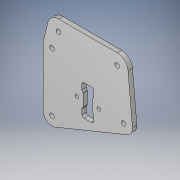
# Autodesk Inventor part: 上昇機構_内側板
Saved by Autodesk Inventor 2019.4 (Build 234330000, 330)
## iProperties
Created: 2021-12-04
Part Number: 上昇機構_内側板
Material: アルミニウム 6061
Document SubType Name: Modeling
Designer: 堀川皓史
Density: 2.7 g/cm^3
Appearance: アルミニウム - フラット
Mass: 27.3834 g
Surface Area: 78.2134 cm^2
Volume: 10.142 cm^3
Author: 堀川皓史
Autodesk Inventor part; units mm, degrees
ref_plane "YZ Plane" through (0, 0, 0) normal (1, 0, 0) x (0, 1, 0)
ref_plane "XZ Plane" through (0, 0, 0) normal (0, 1, 0) x (-1, 0, 0)
ref_plane "XY Plane" through (0, 0, 0) normal (0, 0, 1) x (1, 0, 0)
sketch "スケッチ1" plane through (0, 0, 0) normal (0, 0, 1) x (1, 0, 0)
  line L0 (-15, 61.4764) -> (15, 61.4764) construction
  line L1 (15, 61.4764) -> (15, -42.9448) construction
  line L2 (15, -42.9448) -> (-15, -42.9448) construction
  line L3 (-15, -42.9448) -> (-15, 61.4764) construction
  circle A0 centre (-24.5, 20) radius 9.5 construction
  circle A1 centre (24.5, 0) radius 9.5 construction
  circle A2 centre (-24.5, -20) radius 9.5 construction
  line L4 (-3, 9.5) -> (3, 9.5) construction
  line L5 (3, 9.5) -> (3, -9.5) construction
  line L6 (3, -9.5) -> (-3, -9.5) construction
  line L7 (-3, -9.5) -> (-3, 9.5) construction
  circle A3 centre (-7.5, 0) radius 1.25
  circle A4 centre (7.5, 0) radius 1.25
  circle A5 centre (-20, 32) radius 1.6
  circle A6 centre (20, 32) radius 1.6
  line L8 (-24.5, 20) -> (-24.5, -20) construction
  line L9 (-24.5, -20) -> (24.5, 0) construction
  line L10 (24.5, 0) -> (-24.5, 20) construction
  line L11 (-61.4764, 39.5) -> (49.785, 39.5) construction
  line L12 (49.785, 39.5) -> (49.785, 24.5) construction
  line L13 (49.785, 24.5) -> (-61.4764, 24.5) construction
  line L14 (-61.4764, 24.5) -> (-61.4764, 39.5) construction
  circle A7 centre (-24.5, 20) radius 1.6
  circle A8 centre (24.5, 0) radius 1.6
  circle A9 centre (-24.5, -20) radius 1.6
  arc A10 (-20, 39.5) -> (-27.2824, 33.7934) centre (-20, 32) ccw
  arc A11 (27.4674, 32.6985) -> (20, 39.5) centre (20, 32) ccw
  arc A12 (-30.3259, 21.4347) -> (-30.5, 20) centre (-24.5, 20) ccw
  arc A13 (-30.5, -20) -> (-22.2326, -25.5551) centre (-24.5, -20) ccw
  arc A14 (26.7674, -5.5551) -> (30.4739, 0.5588) centre (24.5, 0) ccw
  line L15 (-20, 39.5) -> (20, 39.5)
  line L16 (-27.2824, 33.7934) -> (-30.3259, 21.4347)
  line L17 (-30.5, 20) -> (-30.5, -20)
  line L18 (-22.2326, -25.5551) -> (26.7674, -5.5551)
  line L19 (30.4739, 0.5588) -> (27.4674, 32.6985)
  line L20 (-2.5, -10.5) -> (2.5, -10.5)
  line L21 (4, -9) -> (4, -5.6703)
  line L22 (2.5, 10.5) -> (-2.5, 10.5)
  line L23 (-3.1, 4) -> (-3.1, -4)
  line L24 (3.1, 4) -> (3.1, -4)
  line L25 (-4, -5.6703) -> (-4, -9)
  line L26 (4, 5.6703) -> (4, 9)
  arc A15 (-2.5, 10.5) -> (-4, 9) centre (-2.5, 9) ccw
  arc A16 (4, 9) -> (2.5, 10.5) centre (2.5, 9) ccw
  arc A17 (-4, -9) -> (-2.5, -10.5) centre (-2.5, -9) ccw
  arc A18 (2.5, -10.5) -> (4, -9) centre (2.5, -9) ccw
  line L27 (-4, 9) -> (-4, 5.6703)
  arc A19 (-4, 5.6703) -> (-3.325, 4.4176) centre (-2.5, 5.6703) ccw
  arc A20 (-3.1, 4) -> (-3.325, 4.4176) centre (-3.6, 4) ccw
  arc A21 (3.325, 4.4176) -> (4, 5.6703) centre (2.5, 5.6703) ccw
  arc A22 (3.325, 4.4176) -> (3.1, 4) centre (3.6, 4) ccw
  arc A23 (-3.325, -4.4176) -> (-4, -5.6703) centre (-2.5, -5.6703) ccw
  arc A24 (-3.325, -4.4176) -> (-3.1, -4) centre (-3.6, -4) ccw
  arc A25 (3.1, -4) -> (3.325, -4.4176) centre (3.6, -4) ccw
  arc A26 (4, -5.6703) -> (3.325, -4.4176) centre (2.5, -5.6703) ccw
  circle A27 centre (-24.5, 20) radius 4 construction
  point P0 (0, 0)
  dimension "d0" = 30
  dimension "d1" = 15
  dimension "d2" = 19
  dimension "d3" = 19
  dimension "d4" = 19
  dimension "d5" = 6
  dimension "d6" = 19
  dimension "d7" = 3
  dimension "d8" = 9.5
  dimension "d9" = 2.5
  dimension "d10" = 2.5
  dimension "d11" = 15
  dimension "d12" = 7.5
  dimension "d13" = 3.2
  dimension "d14" = 3.2
  dimension "d15" = 40
  dimension "d16" = 40
  dimension "d17" = 20
  dimension "d18" = 12
  dimension "d19" = 15
  dimension "d20" = 7.5
  dimension "d21" = 3.2
  dimension "d22" = 3.2
  dimension "d23" = 3.2
  dimension "d24" = 7.5
  dimension "d25" = 7.5
  dimension "d26" = 6
  dimension "d27" = 6
  dimension "d28" = 6
  dimension "d29" = 1
  dimension "d32" = 8
  dimension "d33" = 4
  dimension "d34" = 0.1
  dimension "d35" = 0.1
  dimension "d36" = 1
  dimension "d37" = 1
  dimension "d38" = 1
  dimension "d39" = 1.5
  dimension "d40" = 1
  dimension "d41" = 1.5
  dimension "d42" = 0.5
  dimension "d44" = 1
  dimension "d45" = 1.5
  dimension "d46" = 0.5
  dimension "d47" = 1.5
  dimension "d48" = 0.5
  dimension "d49" = 0.5
  dimension "d50" = 1.5
  dimension "d54" = 8
  constraints: 56 end point, 34 point on circle, 30 tangent, 28 centre point, 9 coincident, 9 parallel, 8 horizontal alignment, 5 perpendicular, 4 horizontal, 3 equal radius, 3 vertical, 2 point on line, 1 equal length
  measures "d0" distance between parallel lines of L1 L3
  measures "d1" distance from line of point (0, 0) L3
  measures "d2" diameter of A0
  measures "d3" diameter of A1
  measures "d4" diameter of A2
  measures "d5" distance of L4.start L4.end
  measures "d6" distance of L4.end L5.end
  measures "d7" distance from line of point (0, 0) L7
  measures "d8" distance from line of point (0, 0) L4
  measures "d9" diameter of A3
  measures "d10" diameter of A4
  measures "d11" distance of A4.centre A3.centre
  measures "d12" distance of point (0, 0) A3.centre
  measures "d13" diameter of A5
  measures "d14" diameter of A6
  measures "d15" distance of L8.end L8.start
  measures "d16" distance of A6.centre A5.centre
  measures "d17" horizontal distance of point (0, 0) A5.centre
  measures "d18" vertical distance of L8.start A5.centre
  measures "d19" distance between parallel lines of L13 L11
  measures "d20" distance from line of A5.centre L13
  measures "d21" diameter of A7
  measures "d22" diameter of A8
  measures "d23" diameter of A9
  measures "d24" radius of A10
  measures "d25" radius of A11
  measures "d26" radius of A12
  measures "d27" radius of A13
  measures "d28" radius of A14
  measures "d29" distance between parallel lines of L6 L20
  measures "d32" distance of L23.start L23.end
  measures "d33" vertical distance of point (0, 0) L23.end
  measures "d34" distance between parallel lines of L23 L7
  measures "d35" distance between parallel lines of L5 L24
  measures "d36" distance between parallel lines of L7 L25
  measures "d37" distance between parallel lines of L5 L21
  measures "d38" distance between parallel lines of L4 L22
  measures "d39" radius of A15
  measures "d40" distance between parallel lines of L7 L27
  measures "d41" radius of A19
  measures "d42" radius of A20
  measures "d44" distance between parallel lines of L5 L26
  measures "d45" radius of A21
  measures "d46" radius of A22
  measures "d47" radius of A23
  measures "d48" radius of A24
  measures "d49" radius of A25
  measures "d50" radius of A26
  measures "d54" diameter of A27
extrude "押し出し1" add sketch "スケッチ1" along normal blind 3
equation "\"d8\" = 0.5 * d6"
equation "\"d12\" = 0.5 * d11"
equation "\"d17\" = 0.5 * d16"
